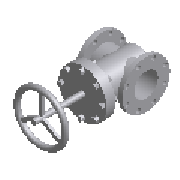
# Autodesk Inventor part: ASME B16.34 Gate Valve Flanged Ends - Class 125 6
Saved by Autodesk Inventor 2020 (Build 240152000, 152)
## iProperties
IsCustomPart: 0
Created: 2018-01-05
Part Number: ASME B16.34 Gate Valve Flanged Ends - Class 125 6
Material: Iron, Cast
Description: Gate Valve
Document SubType Name: Modeling
Standard: ASME B16.34
Designer: alid
Standards Organization: ANSI
Language: en-US
Size Designation: 6
Categories: <MemberInstance><Categories><Category DisplayName="Tube &amp; Pipe" InternalName="4347fa0f-2144-441d-94cd-e3e15c92b736" Mnemonic="TUBEANDPIPE"><CategoryParameter DisplayName="Number of Connections" InternalName="04e9c83a-9e20-4a98-a7e1-e8abe87a2846" Mnemonic="NUM_CONNECTIONS"/><CategoryParameter DisplayName="Angles" InternalName="0e0e4fa4-3bd3-4656-a22e-4e07c8c476f8" Mnemonic="ANGLES"><CategoryParameter DisplayName="Angle" InternalName="9188ad83-1b16-48b4-8b0a-76ce729dafa7" Mnemonic="ANGLE"/></CategoryParameter><CategoryParameter DisplayName="SKey" InternalName="3da84699-049a-4bc2-a65a-6696b77c242f" Mnemonic="SKEY"/><CategoryParameter DisplayName="ISOGEN Description" InternalName="7aa3ba45-b821-4467-8584-f9e6f15f2a7d" Mnemonic="ISOGENDESC"/><CategoryParameter DisplayName="ITEM-CODE" InternalName="99cc3b15-24d9-4d38-aac7-792cfbc57acf" Mnemonic="ITEMCODE"/><CategoryParameter DisplayName="NameOfComponent" InternalName="9c74ad13-48a1-45fe-b0f7-5447561f444a" Mnemonic="NAMEOFCOMPONENT"/><CategoryParameter DisplayName="InLineGroups" InternalName="d60be647-bc43-4c18-a13f-9fe4115f8e64" Mnemonic="INLINEGROUPS"/><Category DisplayName="Fittings" InternalName="ed6b26c4-72b8-4f31-9b63-f85ae8f932e4" Mnemonic="FITTINGS"><CategoryParameter DisplayName="Connections" InternalName="dbd721e8-e885-4eea-9011-b5acfd9f61de" Mnemonic="FIT_CONNECTIONS"><CategoryParameter DisplayName="Min Mating Pipe Size" InternalName="11f51b32-3e37-4310-abf7-f1318a1fd129" Mnemonic="MNMPS"/><CategoryParameter DisplayName="MaxEngagement" InternalName="34fdf028-8797-436e-ba07-ca3dee15bd9b" Mnemonic="MAXENGAGEMENT"/><CategoryParameter DisplayName="NominalSize" InternalName="3f94edc7-e459-48db-8f02-8eebf8cffccd" Mnemonic="NS"/><CategoryParameter DisplayName="DisplayName" InternalName="50f521dd-e050-43f7-9895-6b30ea7ed42e" Mnemonic="DISPLAYNAME"/><CategoryParameter DisplayName="Cut Mating Pipe" InternalName="53a63a6e-53d8-4ca9-8880-037731d1cceb" Mnemonic="CMP"/><CategoryParameter DisplayName="Gender Neutral" InternalName="628bd5f1-acad-44e2-9d91-af996ab74fc2" Mnemonic="NEUTRAL"/><CategoryParameter DisplayName="MinEngagement [% of MaxEngagement]" InternalName="7ec1bde5-73f0-45b1-98d8-365a6c67f8ad" Mnemonic="MINENGAGEMENT"/><CategoryParameter DisplayName="Fixed" InternalName="9142902a-6a8a-446d-9eb8-4b7ce7d245ef" Mnemonic="FIXED"/><CategoryParameter DisplayName="Female" InternalName="b366bcb5-a500-4bad-84bb-22f956216d69" Mnemonic="FEMALE"/><CategoryParameter DisplayName="FlipDirection" InternalName="d55dedc0-f14a-4283-86b4-a4eeb253c8aa" Mnemonic="FLIPDIRECTION"/><CategoryParameter DisplayName="ScheduleNumber" InternalName="d6161c62-eb59-4495-a086-874847c10866" Mnemonic="SN"/><CategoryParameter DisplayName="EndTreatment" InternalName="d7f11516-3374-45ca-b1c7-4b2d63244ae2" Mnemonic="ENDTREATMENT"/><CategoryParameter DisplayName="Max Mating Pipe Size" InternalName="e73ef66b-c04b-45ac-9b32-f712653e25ee" Mnemonic="MXMPS"/></CategoryParameter><CategoryParameter DisplayName="Connections" InternalName="dbd721e8-e885-4eea-9011-b5acfd9f61de" Mnemonic="FIT_CONNECTIONS"><CategoryParameter DisplayName="Min Mating Pipe Size" InternalName="11f51b32-3e37-4310-abf7-f1318a1fd129" Mnemonic="MNMPS"/><CategoryParameter DisplayName="MaxEngagement" InternalName="34fdf028-8797-436e-ba07-ca3dee15bd9b" Mnemonic="MAXENGAGEMENT"/><CategoryParameter DisplayName="NominalSize" InternalName="3f94edc7-e459-48db-8f02-8eebf8cffccd" Mnemonic="NS"/><CategoryParameter DisplayName="DisplayName" InternalName="50f521dd-e050-43f7-9895-6b30ea7ed42e" Mnemonic="DISPLAYNAME"/><CategoryParameter DisplayName="Cut Mating Pipe" InternalName="53a63a6e-53d8-4ca9-8880-037731d1cceb" Mnemonic="CMP"/><CategoryParameter DisplayName="Gender Neutral" InternalName="628bd5f1-acad-44e2-9d91-af996ab74fc2" Mnemonic="NEUTRAL"/><CategoryParameter DisplayName="MinEngagement [% of MaxEngagement]" InternalName="7ec1bde5-73f0-45b1-98d8-365a6c67f8ad" Mnemonic="MINENGAGEMENT"/><CategoryParameter DisplayName="Fixed" InternalName="9142902a-6a8a-446d-9eb8-4b7ce7d245ef" Mnemonic="FIXED"/><CategoryParameter DisplayName="Female" InternalName="b366bcb5-a500-4bad-84bb-22f956216d69" Mnemonic="FEMALE"/><CategoryParameter DisplayName="FlipDirection" InternalName="d55dedc0-f14a-4283-86b4-a4eeb253c8aa" Mnemonic="FLIPDIRECTION"/><CategoryParameter DisplayName="ScheduleNumber" InternalName="d6161c62-eb59-4495-a086-874847c10866" Mnemonic="SN"/><CategoryParameter DisplayName="EndTreatment" InternalName="d7f11516-3374-45ca-b1c7-4b2d63244ae2" Mnemonic="ENDTREATMENT"/><CategoryParameter DisplayName="Max Mating Pipe Size" InternalName="e73ef66b-c04b-45ac-9b32-f712653e25ee" Mnemonic="MXMPS"/></CategoryParameter><Category DisplayName="Valves" InternalName="b54f24b4-8c71-4f76-b075-760a31c67e8e" Mnemonic="Valve"><Category DisplayName="Gate Valves" InternalName="dde97946-8c0f-41b1-aea4-a1b6c9abe529" Mnemonic="Gate_Valve"/></Category></Category></Category><Category DisplayName="DataType" InternalName="23b78d0f-2648-40c6-8793-ca6db495c9e8" Mnemonic="DATATYPE"><CategoryParameter DisplayName="DisplayName" InternalName="05415f3d-3907-474b-a020-eb9d644f4cf3" Mnemonic="DISPLAYNAME"/><CategoryParameter DisplayName="Standard" InternalName="0c0a119c-1e12-4c84-803f-101930972f5e" Mnemonic="STANDARD"/><CategoryParameter DisplayName="Description" InternalName="13903e3d-64b1-4950-80da-f627842ea37f" Mnemonic="DESCRIPTION"/><CategoryParameter DisplayName="Designation" InternalName="2675968c-4ce5-49e0-a4f5-552d29089031" Mnemonic="DESIGNATION"/><CategoryParameter DisplayName="Default Row" InternalName="2af9ec52-faaa-4026-b378-f9fa4afca842" Mnemonic="DEFAULTROW"/><CategoryParameter DisplayName="Folder Name" InternalName="3f06958e-8713-4116-9be7-ed6184ecc97b" Mnemonic="FOLDERNAME"/><CategoryParameter DisplayName="Revision Guid" InternalName="45a75005-10b1-4dfc-8d6d-dfe629f0b93c" Mnemonic="REVISIONGUID"/><CategoryParameter DisplayName="FileName" InternalName="8b46a4cc-9585-4fed-90c3-899f57e09a73" Mnemonic="FILENAME"/><CategoryParameter DisplayName="StdsOrg" InternalName="8f5914e1-4693-403f-8ab5-d37768198c9d" Mnemonic="STDSORG"/><CategoryParameter DisplayName="Family Version" InternalName="914462f6-6e19-4b14-ba84-155b9680b1d0" Mnemonic="FAMILYREVISION"/><CategoryParameter DisplayName="Standard Revision" InternalName="91d5a463-65c2-4fde-b823-3b7fea5e8e17" Mnemonic="STANDARDREVISION"/><CategoryParameter DisplayName="Member Revision" InternalName="a65d44b9-392f-4f4f-857b-e4b3d54996fe" Mnemonic="MEMBERREVISION"/><CategoryParameter DisplayName="ClipFormat" InternalName="bc51e27b-3422-4e78-93ef-cec197ddf230" Mnemonic="CLIPFORMAT"/><CategoryParameter DisplayName="Manufacturer" InternalName="cd6c7a72-a28a-4e50-99a9-2c7f4e13e5ad" Mnemonic="MANUFACTURER"/><CategoryParameter DisplayName="InternalName" InternalName="cf1d0246-76d9-4b4a-8305-fa0409afb5c1" Mnemonic="INTERNALNAME"/><CategoryParameter DisplayName="IsMetric" InternalName="e2385c5b-1ea4-4823-96a8-8de651266ec3" Mnemonic="ISMETRIC"/><Category DisplayName="Part" InternalName="c0e0b642-3bcb-4cc8-9e80-f96d35c4afa4" Mnemonic="PART"><CategoryParameter DisplayName="Part Number" InternalName="016b6077-bfbe-49bd-92c9-d8d59c39c941" Mnemonic="PARTNUMBER"/><CategoryParameter DisplayName="Stock Number" InternalName="4dba7c1c-e26c-444e-836c-b08b433409a8" Mnemonic="STOCKNUMBER"/><CategoryParameter DisplayName="Material Key" InternalName="5c9a8adb-dd2b-4535-b97f-0a94a95fe41f" Mnemonic="MATERIALKEY"/><CategoryParameter DisplayName="Material" InternalName="818a152a-d3c3-49ca-80ee-df7d91421b8e" Mnemonic="MATERIAL"/></Category></Category><Category DisplayName="LegacyMap" InternalName="dfeab48a-acc2-4514-a11c-1b8dc28c3d5f" Mnemonic="LEGACYMAP"><CategoryParameter DisplayName="CatalogID" InternalName="0da51c36-8fd3-4028-86cc-0c9c9e96136a" Mnemonic="CATALOGID"/><CategoryParameter DisplayName="FamilyID" InternalName="1c0b589c-8bbe-4e1e-80cf-07c0de42ac2a" Mnemonic="FAMILYID"/><CategoryParameter DisplayName="MemberID" InternalName="a368ea03-db8a-4d6e-962b-2aa46306b8f5" Mnemonic="MEMBERID"/></Category></Categories><FamilyTemplate Id="ASME B16.34 Gate Valve Flanged Ends - Class 125"><FamilyTemplateParameters><FamilyTemplateParameter ObjectType="kUserParameterObject" ValueType="xs:double" Id="1" ObjectReferenceKey="A"/><FamilyTemplateParameter ObjectType="kUserParameterObject" ValueType="xs:double" Id="2" ObjectReferenceKey="H"/><FamilyTemplateParameter ObjectType="kUserParameterObject" ValueType="xs:double" Id="3" ObjectReferenceKey="D"/><FamilyTemplateParameter ObjectType="kUserParameterObject" ValueType="xs:double" Id="4" ObjectReferenceKey="t"/><FamilyTemplateParameter ObjectType="kUserParameterObject" ValueType="xs:double" Id="5" ObjectReferenceKey="O"/><FamilyTemplateParameter ObjectType="kUserParameterObject" ValueType="xs:double" Id="6" ObjectReferenceKey="C1"/><FamilyTemplateParameter ObjectType="kUserParameterObject" ValueType="xs:double" Id="7" ObjectReferenceKey="BC"/><FamilyTemplateParameter ObjectType="kUserParameterObject" ValueType="xs:double" Id="8" ObjectReferenceKey="DH"/><FamilyTemplateParameter ObjectType="kUserParameterObject" ValueType="xs:integer" Id="9" ObjectReferenceKey="Nu"/><FamilyTemplateParameter ObjectType="kUserParameterObject" ValueType="xs:double" Id="10" ObjectReferenceKey="d"/><FamilyTemplateParameter ObjectType="kUserParameterObject" ValueType="xs:integer" Id="11" ObjectReferenceKey="x"/><FamilyTemplateParameter ObjectType="kUserParameterObject" ValueType="xs:string" Id="121" ObjectReferenceKey="Size_Designation"/><FamilyTemplateParameter ObjectType="kPropertyObject" ValueType="xs:string" Id="100" ObjectReferenceKey="{32853F0F-3444-11d1-9E93-0060B03C1CA6}" SubObjectId="52"/><FamilyTemplateParameter ObjectType="kPropertyObject" ValueType="xs:string" Id="105" ObjectReferenceKey="{32853F0F-3444-11d1-9E93-0060B03C1CA6}" SubObjectId="5"/><FamilyTemplateParameter ObjectType="kPartComponentDefinitionObject" ValueType="xs:string" Id="110" SubObjectId="Material"/></FamilyTemplateParameters></FamilyTemplate><CategoryParameterMap><ParamToTemplateMap><ParamToTemplate CategoryParameter="//CategoryParameter[@InternalName='d60be647-bc43-4c18-a13f-9fe4115f8e64']" ConstantValue="1"/><ParamToTemplate CategoryParameter="//CategoryParameter[@InternalName='04e9c83a-9e20-4a98-a7e1-e8abe87a2846']" ConstantValue="2"/><ParamToTemplate CategoryParameter="//CategoryParameter[@InternalName='0e0e4fa4-3bd3-4656-a22e-4e07c8c476f8']" ConstantValue=""/><ParamToTemplate CategoryParameter="//CategoryParameter[@InternalName='0e0e4fa4-3bd3-4656-a22e-4e07c8c476f8'][1]/CategoryParameter[@InternalName='9188ad83-1b16-48b4-8b0a-76ce729dafa7']" ConstantValue="3.14159265358979"/><ParamToTemplate CategoryParameter="//CategoryParameter[@InternalName='9c74ad13-48a1-45fe-b0f7-5447561f444a']" ConstantValue="VALVE"/><ParamToTemplate CategoryParameter="//CategoryParameter[@InternalName='3da84699-049a-4bc2-a65a-6696b77c242f']" ConstantValue="VTFL"/><ParamToTemplate CategoryParameter="//CategoryParameter[@InternalName='dbd721e8-e885-4eea-9011-b5acfd9f61de'][1]/CategoryParameter[@InternalName='d55dedc0-f14a-4283-86b4-a4eeb253c8aa']" ConstantValue="true"/><ParamToTemplate CategoryParameter="//CategoryParameter[@InternalName='dbd721e8-e885-4eea-9011-b5acfd9f61de'][1]/CategoryParameter[@InternalName='50f521dd-e050-43f7-9895-6b30ea7ed42e']" ConstantValue="Connection1"/><ParamToTemplate CategoryParameter="//CategoryParameter[@InternalName='dbd721e8-e885-4eea-9011-b5acfd9f61de'][1]/CategoryParameter[@InternalName='b366bcb5-a500-4bad-84bb-22f956216d69']" ConstantValue="true"/><ParamToTemplate CategoryParameter="//CategoryParameter[@InternalName='dbd721e8-e885-4eea-9011-b5acfd9f61de'][1]/CategoryParameter[@InternalName='d7f11516-3374-45ca-b1c7-4b2d63244ae2']" ConstantValue="Flanged"/><ParamToTemplate CategoryParameter="//CategoryParameter[@InternalName='dbd721e8-e885-4eea-9011-b5acfd9f61de'][1]/CategoryParameter[@InternalName='9142902a-6a8a-446d-9eb8-4b7ce7d245ef']" ConstantValue="true"/><ParamToTemplate CategoryParameter="//CategoryParameter[@InternalName='dbd721e8-e885-4eea-9011-b5acfd9f61de'][1]/CategoryParameter[@InternalName='34fdf028-8797-436e-ba07-ca3dee15bd9b']" ConstantValue="0"/><ParamToTemplate CategoryParameter="//CategoryParameter[@InternalName='dbd721e8-e885-4eea-9011-b5acfd9f61de'][1]/CategoryParameter[@InternalName='7ec1bde5-73f0-45b1-98d8-365a6c67f8ad']" ConstantValue="0"/><ParamToTemplate CategoryParameter="//CategoryParameter[@InternalName='dbd721e8-e885-4eea-9011-b5acfd9f61de'][2]/CategoryParameter[@InternalName='d55dedc0-f14a-4283-86b4-a4eeb253c8aa']" ConstantValue="false"/><ParamToTemplate CategoryParameter="//CategoryParameter[@InternalName='dbd721e8-e885-4eea-9011-b5acfd9f61de'][2]/CategoryParameter[@InternalName='50f521dd-e050-43f7-9895-6b30ea7ed42e']" ConstantValue="Connection2"/><ParamToTemplate CategoryParameter="//CategoryParameter[@InternalName='dbd721e8-e885-4eea-9011-b5acfd9f61de'][2]/CategoryParameter[@InternalName='b366bcb5-a500-4bad-84bb-22f956216d69']" ConstantValue="true"/><ParamToTemplate CategoryParameter="//CategoryParameter[@InternalName='dbd721e8-e885-4eea-9011-b5acfd9f61de'][2]/CategoryParameter[@InternalName='d7f11516-3374-45ca-b1c7-4b2d63244ae2']" ConstantValue="Flanged"/><ParamToTemplate CategoryParameter="//CategoryParameter[@InternalName='dbd721e8-e885-4eea-9011-b5acfd9f61de'][2]/CategoryParameter[@InternalName='9142902a-6a8a-446d-9eb8-4b7ce7d245ef']" ConstantValue="true"/><ParamToTemplate CategoryParameter="//CategoryParameter[@InternalName='dbd721e8-e885-4eea-9011-b5acfd9f61de'][2]/CategoryParameter[@InternalName='34fdf028-8797-436e-ba07-ca3dee15bd9b']" ConstantValue="0"/><ParamToTemplate CategoryParameter="//CategoryParameter[@InternalName='dbd721e8-e885-4eea-9011-b5acfd9f61de'][2]/CategoryParameter[@InternalName='7ec1bde5-73f0-45b1-98d8-365a6c67f8ad']" ConstantValue="0"/><ParamToTemplate CategoryParameter="//CategoryParameter[@InternalName='dbd721e8-e885-4eea-9011-b5acfd9f61de'][1]/CategoryParameter[@InternalName='628bd5f1-acad-44e2-9d91-af996ab74fc2']" ConstantValue="true"/><ParamToTemplate CategoryParameter="//CategoryParameter[@InternalName='dbd721e8-e885-4eea-9011-b5acfd9f61de'][2]/CategoryParameter[@InternalName='628bd5f1-acad-44e2-9d91-af996ab74fc2']" ConstantValue="true"/><ParamToTemplate CategoryParameter="//CategoryParameter[@InternalName='05415f3d-3907-474b-a020-eb9d644f4cf3']" ConstantValue="ASME B16.34 Gate Valve Flanged Ends - Class 125"/><ParamToTemplate CategoryParameter="//CategoryParameter[@InternalName='cf1d0246-76d9-4b4a-8305-fa0409afb5c1']" ConstantValue="81baf052-bef1-49bc-a63f-52b8a1452a66"/><ParamToTemplate CategoryParameter="//CategoryParameter[@InternalName='3f06958e-8713-4116-9be7-ed6184ecc97b']" ConstantValue="ASME B16.34(23)"/><ParamToTemplate CategoryParameter="//CategoryParameter[@InternalName='914462f6-6e19-4b14-ba84-155b9680b1d0']" ConstantValue="10"/><ParamToTemplate CategoryParameter="//CategoryParameter[@InternalName='13903e3d-64b1-4950-80da-f627842ea37f']" ConstantValue="Gate Valve"/><ParamToTemplate CategoryParameter="//CategoryParameter[@InternalName='8f5914e1-4693-403f-8ab5-d37768198c9d']" ConstantValue="ANSI"/><ParamToTemplate CategoryParameter="//CategoryParameter[@InternalName='0c0a119c-1e12-4c84-803f-101930972f5e']" ConstantValue="ASME B16.34"/><ParamToTemplate CategoryParameter="//CategoryParameter[@InternalName='cd6c7a72-a28a-4e50-99a9-2c7f4e13e5ad']" TemplateParameter="104"/><ParamToTemplate CategoryParameter="//CategoryParameter[@InternalName='91d5a463-65c2-4fde-b823-3b7fea5e8e17']" TemplateParameter="103"/><ParamToTemplate CategoryParameter="//CategoryParameter[@InternalName='bc51e27b-3422-4e78-93ef-cec197ddf230']" ConstantValue="CF_INVENTOR.STDPARTS"/><ParamToTemplate CategoryParameter="//CategoryParameter[@InternalName='e2385c5b-1ea4-4823-96a8-8de651266ec3']" ConstantValue="false"/><ParamToTemplate CategoryParameter="//CategoryParameter[@InternalName='45a75005-10b1-4dfc-8d6d-dfe629f0b93c']" ConstantValue="cd1bb359-03f5-4c9b-b143-be5d1f0c6437"/><ParamToTemplate CategoryParameter="//CategoryParameter[@InternalName='2af9ec52-faaa-4026-b378-f9fa4afca842']" ConstantValue="5"/><ParamToTemplate CategoryParameter="//CategoryParameter[@InternalName='0da51c36-8fd3-4028-86cc-0c9c9e96136a']" ConstantValue="4DA64A5D-C2A1-4499-9EC0-0CCCC70B216C"/><ParamToTemplate CategoryParameter="//CategoryParameter[@InternalName='1c0b589c-8bbe-4e1e-80cf-07c0de42ac2a']" ConstantValue="81baf052-bef1-49bc-a63f-52b8a1452a66"/><ParamToTemplate CategoryParameter="//CategoryParameter[@InternalName='99cc3b15-24d9-4d38-aac7-792cfbc57acf']" ConstantValue=""/><ParamToTemplate CategoryParameter="//CategoryParameter[@InternalName='7aa3ba45-b821-4467-8584-f9e6f15f2a7d']" ConstantValue=""/><ParamToTemplate CategoryParameter="//CategoryParameter[@InternalName='dbd721e8-e885-4eea-9011-b5acfd9f61de'][1]/CategoryParameter[@InternalName='3f94edc7-e459-48db-8f02-8eebf8cffccd']" ConstantValue="6"/><ParamToTemplate CategoryParameter="//CategoryParameter[@InternalName='dbd721e8-e885-4eea-9011-b5acfd9f61de'][2]/CategoryParameter[@InternalName='3f94edc7-e459-48db-8f02-8eebf8cffccd']" ConstantValue="6"/><ParamToTemplate CategoryParameter="//CategoryParameter[@InternalName='8b46a4cc-9585-4fed-90c3-899f57e09a73']" ConstantValue="ASME B16.34 Gate Valve Flanged Ends - Class 125 6"/><ParamToTemplate CategoryParameter="//CategoryParameter[@InternalName='a65d44b9-392f-4f4f-857b-e4b3d54996fe']" ConstantValue="2b43dcef-b75a-442d-a3ee-8b72cfb33dba"/><ParamToTemplate CategoryParameter="//CategoryParameter[@InternalName='a368ea03-db8a-4d6e-962b-2aa46306b8f5']" ConstantValue="5659F275-C68E-4E65-92A1-8643696D2A8E"/><ParamToTemplate CategoryParameter="//CategoryParameter[@InternalName='2675968c-4ce5-49e0-a4f5-552d29089031']" TemplateParameter="100"/><ParamToTemplate CategoryParameter="//CategoryParameter[@InternalName='818a152a-d3c3-49ca-80ee-df7d91421b8e']" TemplateParameter="110"/><ParamToTemplate CategoryParameter="//CategoryParameter[@InternalName='016b6077-bfbe-49bd-92c9-d8d59c39c941']" TemplateParameter="105"/></ParamToTemplateMap></CategoryParameterMap></MemberInstance>
Density: 7.15 g/cm^3
Appearance: Iron Gray
NAME: PIPING: ASME B16.34 Gate Valve Flanged Ends - Class 125
DATA: <meta><inlinegroups number="1" deflen="25.4"></inlinegroups><connections number="2"></connections><angles><a>3.14159265358979</a></angles></meta>
Author: alid
Autodesk Inventor part; units mm, degrees
ref_plane "YZ Plane" through (0, 0, 0) normal (1, 0, 0) x (0, 1, 0)
ref_plane "XZ Plane" through (0, 0, 0) normal (0, 1, 0) x (-1, 0, 0)
sketch "Sketch1" plane through (0, 0, 0) normal (0, 0, 1) x (1, 0, 0)
  line L0 (0, 0) -> (0, 139.7)
  line L1 (0, 139.7) -> (25.4, 139.7)
  line L2 (25.4, 139.7) -> (25.4, 90.424)
  line L3 (25.4, 90.424) -> (241.3, 90.424)
  line L4 (133.35, 90.424) -> (133.35, 0) construction
  line L5 (266.7, 0) -> (0, 0)
  line L6 (266.7, 0) -> (266.7, 139.7)
  line L7 (266.7, 139.7) -> (241.3, 139.7)
  line L8 (241.3, 139.7) -> (241.3, 90.424)
  dimension "d0" = 279.4
  dimension "d1" = 25.4
  dimension "d2" = 266.7
  dimension "d3" = 180.848
  constraints: 18 end point, 6 symmetric about line, 2 coincident, 2 midpoint, 2 parallel, 1 vertical, 3 other
  measures "d0" diameter of L1 L5
  measures "d1" distance between parallel lines of L2 L0
  measures "d2" distance of L5.start L0.start
  measures "d3" diameter of L3 L5
revolve "Revolution1" add sketch "Sketch1" angle 360 about axis through (266.7, 0, 0) along (-1, 0, 0)
sketch "Sketch2" plane through (266.7, 0, 0) normal (1, 0, 0) x (0, 0, -1)
  circle A0 centre (0, 0) radius 120.65 construction
  line L0 (0, 0) -> (-111.4661, 46.1708) construction
  circle A1 centre (-111.4661, 46.1708) radius 11.176
  circle A2 centre (0, 0) radius 139.7 projected
  line L1 (0, 0) -> (-120.65, 0) construction
  dimension "d4" = 241.3
  dimension "d5" = 22.352
  dimension "d42" = 22.5
  constraints: 4 end point, 2 centre point, 2 point on circle, 1 coincident, 1 concentric, 1 horizontal
  measures "d4" diameter of A0
  measures "d5" diameter of A1
  measures "d42" angle of L0 L1
extrude "Extrusion1" cut sketch "Sketch2" against normal through all contours A1
pattern_circular "Circular Pattern1" count 8 over 360 about axis through (133.35, 0, 0) along (1, 0, 0) of "Extrusion1"
sketch "Sketch3" plane through (0, 0, 0) normal (0, 1, 0) x (-1, 0, 0)
  line L0 (-266.7, 139.7) -> (-266.7, -139.7) projected
  line L1 (-266.7, 0) -> (0, 0) construction
  line L2 (-133.35, -119.9896) -> (-133.35, 542.036)
  line L3 (-133.35, 542.036) -> (-118.364, 542.036)
  line L4 (-118.364, 542.036) -> (-118.364, 504.571)
  line L5 (-118.364, 512.064) -> (16.51, 512.064) construction
  arc A0 (-11.4543, 489.585) -> (-11.4543, 504.571) centre (1.524, 497.078) ccw
  line L6 (16.51, 482.092) -> (-118.364, 482.092) construction
  line L7 (-118.364, 489.585) -> (-118.364, 228.6)
  line L8 (-118.364, 228.6) -> (6.35, 228.6)
  line L9 (6.35, 228.6) -> (6.35, 177.8)
  line L10 (6.35, 177.8) -> (-33.8836, 177.8)
  line L11 (-33.8836, 177.8) -> (-33.8836, -90.424)
  line L12 (-133.35, 0) -> (-33.8836, 0)
  line L13 (16.51, 512.064) -> (16.51, 482.092) construction
  line L14 (-118.364, 504.571) -> (-11.4543, 504.571)
  line L15 (1.524, 497.078) -> (-133.35, 497.078) construction
  line L16 (-118.364, 489.585) -> (-11.4543, 489.585)
  arc A1 (-133.35, -119.9896) -> (-33.8836, -90.424) centre (-133.35, 62.1087) ccw
  line L17 (-25.4, -90.424) -> (-241.3, -90.424) projected
  line L18 (0, 139.7) -> (0, -139.7) projected
  dimension "d11" = 198.9328
  dimension "d12" = 279.4
  dimension "d14" = 50.8
  dimension "d15" = 177.8
  dimension "d16" = 299.72
  dimension "d17" = 497.078
  dimension "d18" = 14.986
  dimension "d19" = 29.972
  dimension "d20" = 29.972
  dimension "d21" = 14.986
  dimension "d41" = 29.5656
  constraints: 32 end point, 8 point on line, 6 parallel, 6 perpendicular, 5 point on circle, 3 midpoint, 3 tangent, 2 centre point, 2 symmetric about line, 1 collinear, 1 other
  measures "d11" diameter of L11 L2
  measures "d12" diameter of L9 L2
  measures "d14" distance between parallel lines of L10 L8
  measures "d15" distance between parallel lines of L12 L10
  measures "d16" diameter of L13 L2
  measures "d17" distance from line of L1 L15.start
  measures "d18" radius of A0
  measures "d19" distance between parallel lines of L5 L3
  measures "d20" diameter of L4 L2
  measures "d21" distance between parallel lines of L16 L14
  measures "d41" distance from line of L2.start L17
revolve "Revolution2" add sketch "Sketch3" angle 360 about axis through (133.35, 0, -119.9896) along (0, 0, 1)
sketch "Sketch4" plane through (133.35, 0, 504.571) normal (0, 0, 1) x (1, 0, 0)
  circle A0 centre (0, 0) radius 121.8957 projected
  arc A1 (110.205, -52.0906) -> (9.9907, 121.4856) centre (0, 0) ccw
  arc A2 (14.6688, 3.0672) -> (9.9907, 11.1699) centre (0, 0) ccw
  line L0 (0, 0) -> (0, 121.8957) construction
  line L1 (9.9907, 11.1699) -> (9.9907, 121.4856)
  line L2 (14.6688, 3.0672) -> (110.205, -52.0906)
  circle A3 centre (0, 0) radius 14.986 projected
  line L3 (0, 0) -> (105.5648, -60.9479) construction
  arc A4 (-9.9907, 121.4856) -> (-110.205, -52.0906) centre (0, 0) ccw
  arc A5 (-9.9907, 11.1699) -> (-14.6688, 3.0672) centre (0, 0) ccw
  line L4 (-14.6688, 3.0672) -> (-110.205, -52.0906)
  line L5 (-9.9907, 11.1699) -> (-9.9907, 121.4856)
  arc A6 (-100.2143, -69.395) -> (100.2143, -69.395) centre (0, 0) ccw
  arc A7 (-4.6781, -14.2371) -> (4.6781, -14.2371) centre (0, 0) ccw
  line L6 (4.6781, -14.2371) -> (100.2143, -69.395)
  line L7 (-4.6781, -14.2371) -> (-100.2143, -69.395)
  point P0 (-105.5648, -60.9479)
  point P1 (0, 121.8957)
  point P2 (105.5648, -60.9479)
  point P3 (-105.5648, -60.9479)
  dimension "d22" = 120
  dimension "d23" = 9.9907
  dimension "d25" = 9.9907
  dimension "d34" = 360
  constraints: 18 point on circle, 16 end point, 6 centre point, 6 concentric, 3 coincident, 2 parallel, 1 vertical, 37 other
  measures "d22" angle of L2 L1
  measures "d23" distance between parallel lines of L0 L1
  measures "d25" distance between parallel lines of L3 L2
extrude "Extrusion2" cut sketch "Sketch4" against normal up to next contours A0 L2 A2 L1 | L5 A3 L4 A0 | A0 L7 A3 L6
sketch "Sketch5" plane through (266.7, 0, 0) normal (1, 0, 0) x (0, 0, -1)
  circle A0 centre (0, 0) radius 139.7 projected
  circle A1 centre (0, 0) radius 76.2
  dimension "d28" = 152.4
  constraints: 1 centre point, 1 coincident, 1 concentric
  measures "d28" diameter of A1
extrude "Extrusion3" cut sketch "Sketch5" against normal through all contours A1
ref_plane "Work Plane1" through (133.35, 0, 247.65) normal (0, 0, 1) x (1, 0, 0)
sketch "Sketch6" plane through (133.35, 0, 247.65) normal (0, 0, 1) x (1, 0, 0)
  circle A0 centre (0, 0) radius 120.65 construction
  line L0 (0, 0) -> (120.65, 0) construction
  circle A1 centre (120.65, 0) radius 13.4112 construction
  line L1 (127.3556, -11.6144) -> (113.9444, -11.6144)
  line L2 (113.9444, -11.6144) -> (107.2388, 0)
  line L3 (107.2388, 0) -> (113.9444, 11.6144)
  line L4 (113.9444, 11.6144) -> (127.3556, 11.6144)
  line L5 (127.3556, 11.6144) -> (134.0612, 0)
  line L6 (134.0612, 0) -> (127.3556, -11.6144)
  circle A2 centre (0, 0) radius 139.7 projected
  dimension "d30" = 241.3
  dimension "d31" = 26.8224
  constraints: 14 end point, 2 coincident, 1 horizontal, 1 horizontal alignment, 1 parallel, 17 other
extrude "Extrusion4" add sketch "Sketch6" against normal blind 88.9 contours L1 L2 L3 L4 L5 L6
pattern_circular "Circular Pattern2" count 8 over 360 about axis through (133.35, 0, 203.2) along (0, 0, -1) of "Extrusion4"
equation "\"d0\" = O"
equation "\"d1\" = C1"
equation "\"d2\" = A"
equation "\"d3\" = d + 2 * t"
equation "\"d4\" = BC"
equation "\"d5\" = DH"
equation "\"d12\" = O"
equation "\"d14\" = 2 * C1"
equation "\"d15\" = 0.5 * O + 1.5 * C1"
equation "\"d16\" = D"
equation "\"d17\" = H"
equation "\"d18\" = 0.05 * D"
equation "\"d19\" = 0.1 * D"
equation "\"d20\" = 0.1 * D"
equation "\"d21\" = 0.05 * D"
equation "\"d41\" = -0.6 * t + 0.3 * O - 0.3 * d"
equation "\"d23\" = 0.0333333 * D"
equation "\"d25\" = 0.0333333 * D"
equation "\"d28\" = d"
equation "\"d30\" = BC"
equation "\"d31\" = 1.2 * DH"
equation "\"d35\" = 3.5 * C1"
equation "\"A\" = 266.7"
equation "\"H\" = 497.078"
equation "\"D\" = 299.72"
equation "\"d\" = 152.4"
equation "\"t\" = 14.224"
equation "\"O\" = 279.4"
equation "\"C1\" = 25.4"
equation "\"BC\" = 241.3"
equation "\"DH\" = 22.352"
equation "\"d32\" = 0.75 * C1"
equation "\"x\" = 1.1"
body "Solid1"
